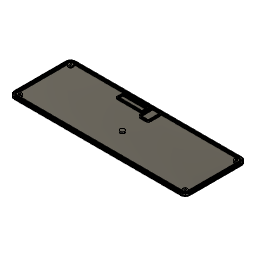
case-bottom (Autodesk Fusion 360 design; units mm, degrees)
Autodesk Fusion 360 part; units mm, degrees
sketch "triplejump-brd" plane through (0, -130, 0) normal (0, 0, 1) x (1, 0, 0)
  spline S0 degree 3 poles (13.4645, 139.4667) (14.4021, 138.529) (15.6739, 138.0022) (17, 138.0022) knots 0 0 0 0 1 1 1 1
  spline S1 degree 3 poles (352, 245.0022) (352, 246.3283) (351.4732, 247.6001) (350.5355, 248.5377) knots 0 0 0 0 1 1 1 1
  spline S2 degree 3 poles (350.5355, 248.5377) (349.5979, 249.4754) (348.3261, 250.0022) (347, 250.0022) knots 0 0 0 0 1 1 1 1
  spline S3 degree 3 poles (12, 143.0022) (12, 141.6761) (12.5268, 140.4043) (13.4645, 139.4667) knots 0 0 0 0 1 1 1 1
  line L0 (17, 138.0022) -> (347, 138.0022)
  spline S4 degree 3 poles (350.5355, 139.4667) (351.4732, 140.4043) (352, 141.6761) (352, 143.0022) knots 0 0 0 0 1 1 1 1
  spline S5 degree 3 poles (17, 250.0022) (15.6739, 250.0022) (14.4021, 249.4754) (13.4645, 248.5377) knots 0 0 0 0 1 1 1 1
  spline S6 degree 3 poles (13.4645, 248.5377) (12.5268, 247.6001) (12, 246.3283) (12, 245.0022) knots 0 0 0 0 1 1 1 1
  line L1 (176, 228.2522) -> (188, 228.2522)
  line L2 (12, 245.0022) -> (12, 143.0022)
  spline S7 degree 3 poles (347, 138.0022) (348.3261, 138.0022) (349.5979, 138.529) (350.5355, 139.4667) knots 0 0 0 0 1 1 1 1
  line L3 (352, 143.0022) -> (352, 245.0022)
  circle A0 centre (17, 245) radius 1.6
  circle A1 centre (17, 143) radius 1.6
  circle A2 centre (347, 143) radius 1.6
  circle A3 centre (347, 245) radius 1.6
  line L4 (166.8312, 244.5585) -> (121.6125, 244.5585)
  line L5 (121.6125, 237.0584) -> (166.8312, 237.0584)
  line L6 (166.8312, 237.0584) -> (166.8312, 244.5585)
  line L7 (121.6125, 244.5585) -> (121.6125, 237.0584)
  line L8 (176, 250.0022) -> (176, 228.2522)
  line L9 (188, 250.0022) -> (188, 228.2522)
  circle A4 centre (17, 245) radius 4.5
  circle A5 centre (17, 143) radius 4.5
  circle A6 centre (347, 143) radius 4.5
  circle A7 centre (347, 245) radius 4.5
  line L10 (277.3601, 186.5709) -> (278.3031, 184.453)
  line L11 (278.3031, 184.453) -> (262.316, 177.3352)
  line L12 (71.141, 245.3466) -> (87.1281, 238.2288)
  line L13 (54.2663, 211.342) -> (38.2793, 218.4598)
  line L14 (38.2793, 218.4598) -> (44.9905, 233.5333)
  line L15 (74.054, 205.1386) -> (55.2349, 213.5173)
  line L16 (89.0724, 195.8453) -> (73.0854, 202.9631)
  line L17 (95.7836, 210.9188) -> (89.0724, 195.8453)
  line L18 (316.9956, 238.0568) -> (334.3986, 245.8051)
  line L19 (297.7067, 234.5441) -> (315.1097, 242.2924)
  line L20 (315.1097, 242.2924) -> (316.9956, 238.0568)
  line L21 (281.7197, 227.4262) -> (280.7767, 229.5441)
  line L22 (296.7638, 236.6619) -> (297.7067, 234.5441)
  line L23 (280.7767, 229.5441) -> (296.7638, 236.6619)
  line L24 (264.3166, 219.6779) -> (281.7197, 227.4262)
  line L25 (265.2595, 217.56) -> (264.3166, 219.6779)
  line L26 (247.8565, 209.8117) -> (265.2595, 217.56)
  line L27 (348.8581, 213.3285) -> (332.8711, 206.2107)
  line L28 (332.8711, 206.2107) -> (330.9852, 210.4463)
  line L29 (313.5822, 202.698) -> (312.6393, 204.8158)
  line L30 (330.9852, 210.4463) -> (313.5822, 202.698)
  line L31 (312.6393, 204.8158) -> (293.8202, 196.437)
  line L32 (294.7632, 194.3192) -> (277.3601, 186.5709)
  line L33 (293.8202, 196.437) -> (294.7632, 194.3192)
  line L34 (83.663, 151.7163) -> (105.102, 167.2926)
  line L35 (105.102, 167.2926) -> (114.8005, 153.9439)
  line L36 (114.8005, 153.9439) -> (93.3615, 138.3676)
  line L37 (93.3615, 138.3676) -> (83.663, 151.7163)
  line L38 (258.898, 167.2926) -> (280.337, 151.7163)
  line L39 (249.1995, 153.9439) -> (258.898, 167.2926)
  line L40 (270.6385, 138.3676) -> (249.1995, 153.9439)
  line L41 (280.337, 151.7163) -> (270.6385, 138.3676)
  line L42 (176, 250.0022) -> (188, 250.0022)
  line L43 (347, 251.0022) -> (188, 251.0022)
  line L44 (176, 251.0022) -> (188, 251.0022)
  line L45 (17, 251.0022) -> (176, 251.0022)
  spline S8 degree 3 poles (17, 251.0022) (15.4091, 251.0022) (13.8823, 250.3698) (12.7574, 249.2448) knots 0 0 0 0 1 1 1 1
  spline S9 degree 3 poles (12.7574, 249.2448) (11.6324, 248.1199) (11, 246.5931) (11, 245.0022) knots 0 0 0 0 1 1 1 1
  line L46 (11, 245.0022) -> (11, 143.0022)
  spline S10 degree 3 poles (11, 143.0022) (11, 141.4113) (11.6324, 139.8845) (12.7574, 138.7596) knots 0 0 0 0 1 1 1 1
  spline S11 degree 3 poles (12.7574, 138.7596) (13.8823, 137.6346) (15.4091, 137.0022) (17, 137.0022) knots 0 0 0 0 1 1 1 1
  line L47 (17, 137.0022) -> (347, 137.0022)
  spline S12 degree 3 poles (347, 137.0022) (348.5909, 137.0022) (350.1177, 137.6346) (351.2426, 138.7596) knots 0 0 0 0 1 1 1 1
  spline S13 degree 3 poles (351.2426, 138.7596) (352.3676, 139.8845) (353, 141.4113) (353, 143.0022) knots 0 0 0 0 1 1 1 1
  line L48 (353, 143.0022) -> (353, 245.0022)
  spline S14 degree 3 poles (353, 245.0022) (353, 246.5931) (352.3676, 248.1199) (351.2426, 249.2448) knots 0 0 0 0 1 1 1 1
  spline S15 degree 3 poles (351.2426, 249.2448) (350.1177, 250.3698) (348.5909, 251.0022) (347, 251.0022) knots 0 0 0 0 1 1 1 1
  line L49 (347, 253.0022) -> (188, 253.0022)
  line L50 (176, 253.0022) -> (188, 253.0022)
  line L51 (17, 253.0022) -> (176, 253.0022)
  spline S16 degree 3 poles (17, 253.0022) (14.8794, 253.0022) (12.8426, 252.1585) (11.3431, 250.6591) knots 0 0 0 0 1 1 1 1
  spline S17 degree 3 poles (11.3431, 250.6591) (9.8437, 249.1596) (9, 247.1228) (9, 245.0022) knots 0 0 0 0 1 1 1 1
  line L52 (9, 245.0022) -> (9, 143.0022)
  spline S18 degree 3 poles (9, 143.0022) (9, 140.8816) (9.8437, 138.8448) (11.3431, 137.3453) knots 0 0 0 0 1 1 1 1
  spline S19 degree 3 poles (11.3431, 137.3453) (12.8426, 135.8459) (14.8794, 135.0022) (17, 135.0022) knots 0 0 0 0 1 1 1 1
  line L53 (17, 135.0022) -> (347, 135.0022)
  spline S20 degree 3 poles (347, 135.0022) (349.1206, 135.0022) (351.1574, 135.8459) (352.6569, 137.3453) knots 0 0 0 0 1 1 1 1
  spline S21 degree 3 poles (352.6569, 137.3453) (354.1563, 138.8448) (355, 140.8816) (355, 143.0022) knots 0 0 0 0 1 1 1 1
  line L54 (355, 143.0022) -> (355, 245.0022)
  spline S22 degree 3 poles (355, 245.0022) (355, 247.1228) (354.1563, 249.1596) (352.6569, 250.6591) knots 0 0 0 0 1 1 1 1
  spline S23 degree 3 poles (352.6569, 250.6591) (351.1574, 252.1585) (349.1206, 253.0022) (347, 253.0022) knots 0 0 0 0 1 1 1 1
  line L55 (347, 255.0022) -> (188, 255.0022)
  line L56 (176, 255.0022) -> (188, 255.0022)
  line L57 (17, 255.0022) -> (176, 255.0022)
  spline S24 degree 3 poles (17, 255.0022) (14.3498, 255.0022) (11.8029, 253.9473) (9.9289, 252.0733) knots 0 0 0 0 1 1 1 1
  spline S25 degree 3 poles (9.9289, 252.0733) (8.0549, 250.1993) (7, 247.6524) (7, 245.0022) knots 0 0 0 0 1 1 1 1
  line L58 (7, 245.0022) -> (7, 143.0022)
  spline S26 degree 3 poles (7, 143.0022) (7, 140.352) (8.0549, 137.8051) (9.9289, 135.9311) knots 0 0 0 0 1 1 1 1
  spline S27 degree 3 poles (9.9289, 135.9311) (11.8029, 134.0571) (14.3498, 133.0022) (17, 133.0022) knots 0 0 0 0 1 1 1 1
  line L59 (17, 133.0022) -> (347, 133.0022)
  spline S28 degree 3 poles (347, 133.0022) (349.6502, 133.0022) (352.1971, 134.0571) (354.0711, 135.9311) knots 0 0 0 0 1 1 1 1
  spline S29 degree 3 poles (354.0711, 135.9311) (355.9451, 137.8051) (357, 140.352) (357, 143.0022) knots 0 0 0 0 1 1 1 1
  line L60 (357, 143.0022) -> (357, 245.0022)
  spline S30 degree 3 poles (357, 245.0022) (357, 247.6524) (355.9451, 250.1993) (354.0711, 252.0733) knots 0 0 0 0 1 1 1 1
  spline S31 degree 3 poles (354.0711, 252.0733) (352.1971, 253.9473) (349.6502, 255.0022) (347, 255.0022) knots 0 0 0 0 1 1 1 1
  line L61 (55.2349, 213.5173) -> (54.2663, 211.342)
  line L62 (71.141, 245.3466) -> (62.3935, 225.785)
  line L63 (87.1281, 238.2288) -> (78.3805, 218.6671)
  line L64 (74.054, 205.1386) -> (73.0854, 202.9631)
  line L65 (44.9905, 233.5333) -> (62.3935, 225.785)
  line L66 (78.3805, 218.6671) -> (95.7836, 210.9188)
  line L67 (247.8565, 209.8117) -> (262.316, 177.3352)
  line L68 (348.8581, 213.3285) -> (334.3986, 245.8051)
  circle A8 centre (182, 183.1272) radius 4.5
  line L69 (350.1754, 143) -> (348.5877, 145.75)
  line L70 (348.5877, 145.75) -> (345.4123, 145.75)
  line L71 (345.4123, 145.75) -> (343.8246, 143)
  line L72 (343.8246, 143) -> (345.4123, 140.25)
  line L73 (345.4123, 140.25) -> (348.5877, 140.25)
  line L74 (348.5877, 140.25) -> (350.1754, 143)
  line L75 (20.1754, 245) -> (18.5877, 247.75)
  line L76 (15.4123, 247.75) -> (13.8246, 245)
  line L77 (18.5877, 247.75) -> (15.4123, 247.75)
  line L78 (18.5877, 242.25) -> (20.1754, 245)
  line L79 (15.4123, 242.25) -> (18.5877, 242.25)
  line L80 (13.8246, 245) -> (15.4123, 242.25)
  line L81 (15.4123, 140.25) -> (18.5877, 140.25)
  line L82 (18.5877, 145.75) -> (15.4123, 145.75)
  line L83 (20.1754, 143) -> (18.5877, 145.75)
  line L84 (15.4123, 145.75) -> (13.8246, 143)
  line L85 (13.8246, 143) -> (15.4123, 140.25)
  line L86 (18.5877, 140.25) -> (20.1754, 143)
  line L87 (348.5877, 242.25) -> (350.1754, 245)
  line L88 (348.5877, 247.75) -> (345.4123, 247.75)
  line L89 (345.4123, 247.75) -> (343.8246, 245)
  line L90 (345.4123, 242.25) -> (348.5877, 242.25)
  line L91 (350.1754, 245) -> (348.5877, 247.75)
  line L92 (343.8246, 245) -> (345.4123, 242.25)
  line L93 (174, 249.0022) -> (174, 228.2522)
  line L94 (176, 226.2522) -> (188, 226.2522)
  line L95 (190, 249.0022) -> (190, 228.2522)
  line L96 (121.6125, 236.0584) -> (166.8312, 236.0584)
  line L97 (167.8312, 237.0584) -> (167.8312, 244.5585)
  line L98 (166.8312, 245.5585) -> (121.6125, 245.5585)
  line L99 (120.6125, 244.5585) -> (120.6125, 237.0584)
  line L100 (44.8904, 235.7672) -> (60.4708, 228.8303)
  line L101 (69.7228, 247.0745) -> (61.7904, 229.3357)
  line L102 (71.0424, 247.5798) -> (88.8566, 239.6484)
  line L103 (89.3627, 238.3267) -> (81.433, 220.5938)
  line L104 (81.9391, 219.272) -> (97.5106, 212.3391)
  line L105 (98.0174, 211.0188) -> (90.4928, 194.1182)
  line L106 (89.1725, 193.6114) -> (71.3584, 201.5428)
  line L107 (71.0067, 203.2114) -> (70.8516, 202.8631)
  line L108 (70.4998, 204.5317) -> (57.1621, 210.47)
  line L109 (55.8418, 209.9632) -> (55.6867, 209.6149)
  line L110 (54.3664, 209.1081) -> (36.5523, 217.0395)
  line L111 (36.0455, 218.3598) -> (43.5701, 235.2604)
  line L112 (116.785, 152.9136) -> (93.7281, 136.1617)
  line L113 (92.3313, 136.383) -> (81.4572, 151.3498)
  line L114 (81.6785, 152.7466) -> (104.7354, 169.4985)
  line L115 (106.1322, 169.2772) -> (117.0063, 154.3104)
  line L116 (299.6339, 237.5914) -> (315.2098, 244.5263)
  line L117 (316.5301, 244.0195) -> (317.6025, 241.6109)
  line L118 (318.9227, 241.1041) -> (334.4987, 248.0389)
  line L119 (351.0919, 213.2285) -> (335.8189, 247.5321)
  line L120 (350.5851, 211.9082) -> (332.771, 203.9768)
  line L121 (331.4507, 204.4836) -> (330.3784, 206.8922)
  line L122 (329.0581, 207.399) -> (313.4821, 200.4641)
  line L123 (312.1618, 200.9709) -> (312.0324, 201.2617)
  line L124 (310.7121, 201.7685) -> (297.3743, 195.8301)
  line L125 (296.8675, 194.5099) -> (296.997, 194.2191)
  line L126 (296.4902, 192.8988) -> (280.9142, 185.964)
  line L127 (280.4074, 184.6437) -> (280.5369, 184.353)
  line L128 (280.0301, 183.0327) -> (262.2159, 175.1013)
  line L129 (245.6227, 209.9118) -> (260.8957, 175.6081)
  line L130 (246.1295, 211.2321) -> (261.7054, 218.1669)
  line L131 (262.2122, 219.4872) -> (262.0828, 219.7779)
  line L132 (262.5896, 221.0982) -> (278.1656, 228.0331)
  line L133 (278.6724, 229.3534) -> (278.5429, 229.6441)
  line L134 (279.0497, 230.9644) -> (296.8639, 238.8958)
  line L135 (298.1841, 238.389) -> (298.3136, 238.0982)
  line L136 (270.2719, 136.1617) -> (247.215, 152.9136)
  line L137 (246.9937, 154.3104) -> (257.8678, 169.2772)
  line L138 (259.2646, 169.4985) -> (282.3215, 152.7466)
  line L139 (282.5428, 151.3498) -> (271.6687, 136.383)
  line L140 (172, 249.0022) -> (172, 228.2522)
  line L141 (176, 224.2522) -> (188, 224.2522)
  line L142 (192, 249.0022) -> (192, 228.2522)
  arc A9 (174, 228.2522) -> (176, 226.2522) centre (176, 228.2522) ccw
  arc A10 (188, 226.2522) -> (190, 228.2522) centre (188, 228.2522) ccw
  arc A11 (174, 249.0022) -> (173, 250.0022) centre (173, 249.0022) ccw
  arc A12 (173, 250.0022) -> (172, 249.0022) centre (173, 249.0022) ccw
  arc A13 (191, 250.0022) -> (190, 249.0022) centre (191, 249.0022) ccw
  arc A14 (192, 249.0022) -> (191, 250.0022) centre (191, 249.0022) ccw
  arc A15 (172, 228.2522) -> (176, 224.2522) centre (176, 228.2522) ccw
  arc A16 (188, 224.2522) -> (192, 228.2522) centre (188, 228.2522) ccw
  line L143 (119.6125, 234.0584) -> (168.8312, 234.0584)
  line L144 (169.8312, 235.0584) -> (169.8312, 246.5585)
  line L145 (168.8312, 247.5585) -> (119.6125, 247.5585)
  line L146 (118.6125, 246.5585) -> (118.6125, 235.0584)
  line L147 (68.7121, 249.7137) -> (60.7798, 231.9749)
  line L148 (43.8768, 238.4077) -> (59.4601, 231.4696)
  line L149 (33.4049, 217.3462) -> (42.5565, 237.9009)
  line L150 (55.38, 206.4676) -> (33.9117, 216.0259)
  line L151 (56.8554, 207.3227) -> (56.7003, 206.9744)
  line L152 (67.8593, 203.5181) -> (58.1757, 207.8295)
  line L153 (68.3661, 202.1978) -> (68.211, 201.8495)
  line L154 (90.1861, 190.9709) -> (68.7178, 200.5292)
  line L155 (100.658, 212.0324) -> (91.5064, 191.4777)
  line L156 (84.5826, 220.2843) -> (100.1512, 213.3527)
  line L157 (92.0062, 239.339) -> (84.0765, 221.6061)
  line L158 (70.0318, 250.2191) -> (91.5001, 240.6607)
  line L159 (259.949, 222.1118) -> (275.525, 229.0467)
  line L160 (276.0318, 230.367) -> (275.9024, 230.6577)
  line L161 (276.4092, 231.978) -> (297.8775, 241.5363)
  line L162 (299.1978, 241.0295) -> (299.3272, 240.7388)
  line L163 (300.6475, 240.232) -> (316.2234, 247.1668)
  line L164 (317.5437, 246.66) -> (318.6161, 244.2515)
  line L165 (319.9364, 243.7446) -> (335.5123, 250.6795)
  line L166 (353.7325, 212.2149) -> (336.8326, 250.1727)
  line L167 (353.2257, 210.8946) -> (331.7574, 201.3363)
  line L168 (330.4371, 201.8431) -> (329.3647, 204.2516)
  line L169 (328.0445, 204.7584) -> (312.4685, 197.8236)
  line L170 (311.1482, 198.3304) -> (311.0188, 198.6211)
  line L171 (309.6985, 199.1279) -> (300.0149, 194.8165)
  line L172 (299.5081, 193.4962) -> (299.6375, 193.2055)
  line L173 (299.1307, 191.8852) -> (283.5548, 184.9504)
  line L174 (283.048, 183.6301) -> (283.1774, 183.3394)
  line L175 (282.6706, 182.0191) -> (261.2023, 172.4608)
  line L176 (242.9821, 210.9254) -> (259.882, 172.9676)
  line L177 (243.4889, 212.2457) -> (259.0648, 219.1805)
  line L178 (259.5717, 220.5008) -> (259.4422, 220.7915)
  line L179 (119.5786, 152.4712) -> (93.2856, 133.3681)
  line L180 (91.8888, 133.5894) -> (78.6636, 151.7922)
  line L181 (78.8849, 153.189) -> (105.1779, 172.2921)
  line L182 (106.5747, 172.0708) -> (119.7999, 153.868)
  line L183 (285.3364, 151.7922) -> (272.1112, 133.5894)
  line L184 (270.7144, 133.3681) -> (244.4214, 152.4712)
  line L185 (244.2001, 153.868) -> (257.4253, 172.0708)
  line L186 (258.8221, 172.2921) -> (285.1151, 153.189)
  arc A17 (43.8768, 238.4077) -> (42.5565, 237.9009) centre (43.47, 237.4942) ccw
  arc A18 (44.8904, 235.7672) -> (43.5701, 235.2604) centre (44.4836, 234.8536) ccw
  arc A19 (59.4601, 231.4696) -> (60.7798, 231.9749) centre (59.8669, 232.3831) ccw
  arc A20 (60.4708, 228.8303) -> (61.7904, 229.3357) centre (60.8775, 229.7439) ccw
  arc A21 (71.0424, 247.5798) -> (69.7228, 247.0745) centre (70.6357, 246.6663) ccw
  arc A22 (70.0318, 250.2191) -> (68.7121, 249.7137) centre (69.625, 249.3055) ccw
  arc A23 (89.3627, 238.3267) -> (88.8566, 239.6484) centre (88.4498, 238.7349) ccw
  arc A24 (92.0062, 239.339) -> (91.5001, 240.6607) centre (91.0934, 239.7472) ccw
  arc A25 (84.0765, 221.6061) -> (84.5826, 220.2843) centre (84.9894, 221.1978) ccw
  arc A26 (81.433, 220.5938) -> (81.9391, 219.272) centre (82.3458, 220.1855) ccw
  arc A27 (100.658, 212.0324) -> (100.1512, 213.3527) centre (99.7444, 212.4392) ccw
  arc A28 (98.0174, 211.0188) -> (97.5106, 212.3391) centre (97.1039, 211.4256) ccw
  arc A29 (89.1725, 193.6114) -> (90.4928, 194.1182) centre (89.5793, 194.525) ccw
  arc A30 (90.1861, 190.9709) -> (91.5064, 191.4777) centre (90.5929, 191.8844) ccw
  arc A31 (70.8516, 202.8631) -> (71.3584, 201.5428) centre (71.7651, 202.4563) ccw
  arc A32 (71.0067, 203.2114) -> (70.4998, 204.5317) centre (70.0931, 203.6181) ccw
  arc A33 (68.3661, 202.1978) -> (67.8593, 203.5181) centre (67.4525, 202.6045) ccw
  arc A34 (68.211, 201.8495) -> (68.7178, 200.5292) centre (69.1246, 201.4427) ccw
  arc A35 (57.1621, 210.47) -> (55.8418, 209.9632) centre (56.7553, 209.5565) ccw
  arc A36 (54.3664, 209.1081) -> (55.6867, 209.6149) centre (54.7732, 210.0217) ccw
  arc A37 (58.1757, 207.8295) -> (56.8554, 207.3227) centre (57.7689, 206.9159) ccw
  arc A38 (55.38, 206.4676) -> (56.7003, 206.9744) centre (55.7868, 207.3811) ccw
  arc A39 (36.0455, 218.3598) -> (36.5523, 217.0395) centre (36.959, 217.953) ccw
  arc A40 (33.4049, 217.3462) -> (33.9117, 216.0259) centre (34.3185, 216.9394) ccw
  arc A41 (121.6125, 245.5585) -> (120.6125, 244.5585) centre (121.6125, 244.5585) ccw
  arc A42 (120.6125, 237.0584) -> (121.6125, 236.0584) centre (121.6125, 237.0584) ccw
  arc A43 (119.6125, 247.5585) -> (118.6125, 246.5585) centre (119.6125, 246.5585) ccw
  arc A44 (118.6125, 235.0584) -> (119.6125, 234.0584) centre (119.6125, 235.0584) ccw
  arc A45 (168.8312, 234.0584) -> (169.8312, 235.0584) centre (168.8312, 235.0584) ccw
  arc A46 (166.8312, 236.0584) -> (167.8312, 237.0584) centre (166.8312, 237.0584) ccw
  arc A47 (167.8312, 244.5585) -> (166.8312, 245.5585) centre (166.8312, 244.5585) ccw
  arc A48 (169.8312, 246.5585) -> (168.8312, 247.5585) centre (168.8312, 246.5585) ccw
  arc A49 (243.4889, 212.2457) -> (242.9821, 210.9254) centre (243.8957, 211.3321) ccw
  arc A50 (246.1295, 211.2321) -> (245.6227, 209.9118) centre (246.5362, 210.3185) ccw
  arc A51 (259.0648, 219.1805) -> (259.5717, 220.5008) centre (258.6581, 220.0941) ccw
  arc A52 (259.949, 222.1118) -> (259.4422, 220.7915) centre (260.3558, 221.1983) ccw
  arc A53 (261.7054, 218.1669) -> (262.2122, 219.4872) centre (261.2987, 219.0805) ccw
  arc A54 (262.5896, 221.0982) -> (262.0828, 219.7779) centre (262.9963, 220.1847) ccw
  arc A55 (275.525, 229.0467) -> (276.0318, 230.367) centre (275.1183, 229.9602) ccw
  arc A56 (276.4092, 231.978) -> (275.9024, 230.6577) centre (276.8159, 231.0645) ccw
  arc A57 (278.1656, 228.0331) -> (278.6724, 229.3534) centre (277.7588, 228.9466) ccw
  arc A58 (279.0497, 230.9644) -> (278.5429, 229.6441) centre (279.4565, 230.0509) ccw
  arc A59 (299.1978, 241.0295) -> (297.8775, 241.5363) centre (298.2842, 240.6228) ccw
  arc A60 (298.1841, 238.389) -> (296.8639, 238.8958) centre (297.2706, 237.9822) ccw
  arc A61 (298.3136, 238.0982) -> (299.6339, 237.5914) centre (299.2271, 238.505) ccw
  arc A62 (299.3272, 240.7388) -> (300.6475, 240.232) centre (300.2408, 241.1455) ccw
  arc A63 (316.5301, 244.0195) -> (315.2098, 244.5263) centre (315.6166, 243.6127) ccw
  arc A64 (317.5437, 246.66) -> (316.2234, 247.1668) centre (316.6302, 246.2533) ccw
  arc A65 (318.6161, 244.2515) -> (319.9364, 243.7446) centre (319.5296, 244.6582) ccw
  arc A66 (317.6025, 241.6109) -> (318.9227, 241.1041) centre (318.516, 242.0176) ccw
  arc A67 (336.8326, 250.1727) -> (335.5123, 250.6795) centre (335.919, 249.7659) ccw
  arc A68 (335.8189, 247.5321) -> (334.4987, 248.0389) centre (334.9054, 247.1254) ccw
  arc A69 (353.2257, 210.8946) -> (353.7325, 212.2149) centre (352.8189, 211.8081) ccw
  arc A70 (350.5851, 211.9082) -> (351.0919, 213.2285) centre (350.1784, 212.8217) ccw
  arc A71 (331.4507, 204.4836) -> (332.771, 203.9768) centre (332.3642, 204.8904) ccw
  arc A72 (330.4371, 201.8431) -> (331.7574, 201.3363) centre (331.3506, 202.2498) ccw
  arc A73 (330.3784, 206.8922) -> (329.0581, 207.399) centre (329.4648, 206.4854) ccw
  arc A74 (329.3647, 204.2516) -> (328.0445, 204.7584) centre (328.4512, 203.8449) ccw
  arc A75 (312.1618, 200.9709) -> (313.4821, 200.4641) centre (313.0754, 201.3777) ccw
  arc A76 (311.1482, 198.3304) -> (312.4685, 197.8236) centre (312.0618, 198.7371) ccw
  arc A77 (312.0324, 201.2617) -> (310.7121, 201.7685) centre (311.1188, 200.855) ccw
  arc A78 (311.0188, 198.6211) -> (309.6985, 199.1279) centre (310.1052, 198.2144) ccw
  arc A79 (297.3743, 195.8301) -> (296.8675, 194.5099) centre (297.7811, 194.9166) ccw
  arc A80 (296.4902, 192.8988) -> (296.997, 194.2191) centre (296.0834, 193.8124) ccw
  arc A81 (300.0149, 194.8165) -> (299.5081, 193.4962) centre (300.4216, 193.903) ccw
  arc A82 (299.1307, 191.8852) -> (299.6375, 193.2055) centre (298.724, 192.7988) ccw
  arc A83 (280.9142, 185.964) -> (280.4074, 184.6437) centre (281.321, 185.0504) ccw
  arc A84 (280.0301, 183.0327) -> (280.5369, 184.353) centre (279.6233, 183.9462) ccw
  arc A85 (283.5548, 184.9504) -> (283.048, 183.6301) centre (283.9615, 184.0368) ccw
  arc A86 (282.6706, 182.0191) -> (283.1774, 183.3394) centre (282.2639, 182.9326) ccw
  arc A87 (260.8957, 175.6081) -> (262.2159, 175.1013) centre (261.8092, 176.0149) ccw
  arc A88 (259.882, 172.9676) -> (261.2023, 172.4608) centre (260.7956, 173.3743) ccw
  line L187 (17, 250.0022) -> (347, 250.0022)
  arc A89 (259.2646, 169.4985) -> (257.8678, 169.2772) centre (258.6768, 168.6894) ccw
  arc A90 (258.8221, 172.2921) -> (257.4253, 172.0708) centre (258.2343, 171.4831) ccw
  arc A91 (285.3364, 151.7922) -> (285.1151, 153.189) centre (284.5274, 152.38) ccw
  arc A92 (282.5428, 151.3498) -> (282.3215, 152.7466) centre (281.7338, 151.9376) ccw
  arc A93 (270.2719, 136.1617) -> (271.6687, 136.383) centre (270.8597, 136.9708) ccw
  arc A94 (270.7144, 133.3681) -> (272.1112, 133.5894) centre (271.3022, 134.1771) ccw
  arc A95 (246.9937, 154.3104) -> (247.215, 152.9136) centre (247.8027, 153.7226) ccw
  arc A96 (244.2001, 153.868) -> (244.4214, 152.4712) centre (245.0091, 153.2802) ccw
  arc A97 (81.6785, 152.7466) -> (81.4572, 151.3498) centre (82.2662, 151.9376) ccw
  arc A98 (92.3313, 136.383) -> (93.7281, 136.1617) centre (93.1403, 136.9708) ccw
  arc A99 (106.1322, 169.2772) -> (104.7354, 169.4985) centre (105.3232, 168.6894) ccw
  arc A100 (116.785, 152.9136) -> (117.0063, 154.3104) centre (116.1973, 153.7226) ccw
  arc A101 (106.5747, 172.0708) -> (105.1779, 172.2921) centre (105.7657, 171.4831) ccw
  arc A102 (119.5786, 152.4712) -> (119.7999, 153.868) centre (118.9909, 153.2802) ccw
  arc A103 (78.8849, 153.189) -> (78.6636, 151.7922) centre (79.4726, 152.38) ccw
  arc A104 (91.8888, 133.5894) -> (93.2856, 133.3681) centre (92.6978, 134.1771) ccw
  line L188 (175.5, 255.0022) -> (188.5, 255.0022)
  line L189 (188.5, 255.0022) -> (188.5, 250.0022)
  line L190 (188.5, 250.0022) -> (175.5, 250.0022)
  line L191 (175.5, 250.0022) -> (175.5, 255.0022)
  point P0 (182, 183.1272)
  point P1 (347, 143)
  point P2 (17, 245)
  point P3 (17, 143)
  point P4 (347, 245)
  point P5 (182, 255.0022)
  point P6 (182, 255.0022)
  dimension "d90" = 3.1754
  dimension "d91" = 3.1754
  dimension "d92" = 3.1754
  dimension "d93" = 3.1754
  dimension "d112" = 2
  dimension "d113" = 2
  dimension "d114" = 1
  dimension "d115" = 1
  dimension "d116" = 1
  dimension "d117" = 1
  dimension "d118" = 4
  dimension "d119" = 4
  dimension "d125" = 1
  dimension "d126" = 1
  dimension "d127" = 1
  dimension "d128" = 1
  dimension "d129" = 1
  dimension "d130" = 1
  dimension "d131" = 1
  dimension "d132" = 1
  dimension "d133" = 1
  dimension "d134" = 1
  dimension "d135" = 1
  dimension "d136" = 1
  dimension "d137" = 1
  dimension "d138" = 1
  dimension "d139" = 1
  dimension "d140" = 1
  dimension "d141" = 1
  dimension "d142" = 1
  dimension "d143" = 1
  dimension "d144" = 1
  dimension "d145" = 1
  dimension "d146" = 1
  dimension "d147" = 1
  dimension "d148" = 1
  dimension "d149" = 1
  dimension "d150" = 1
  dimension "d151" = 1
  dimension "d152" = 1
  dimension "d153" = 1
  dimension "d154" = 1
  dimension "d155" = 1
  dimension "d156" = 1
  dimension "d157" = 1
  dimension "d158" = 1
  dimension "d159" = 1
  dimension "d160" = 1
  dimension "d161" = 1
  dimension "d162" = 1
  dimension "d163" = 1
  dimension "d164" = 1
  dimension "d165" = 1
  dimension "d166" = 1
  dimension "d167" = 1
  dimension "d168" = 1
  dimension "d169" = 1
  dimension "d170" = 1
  dimension "d171" = 1
  dimension "d172" = 1
  dimension "d173" = 1
  dimension "d174" = 1
  dimension "d175" = 1
  dimension "d176" = 1
  dimension "d177" = 1
  dimension "d178" = 1
  dimension "d179" = 1
  dimension "d180" = 1
  dimension "d181" = 1
  dimension "d182" = 1
  dimension "d183" = 1
  dimension "d184" = 1
  dimension "d185" = 1
  dimension "d186" = 1
  dimension "d187" = 1
  dimension "d188" = 1
  dimension "d189" = 1
  dimension "d190" = 1
  dimension "d191" = 1
  dimension "d192" = 1
  dimension "d193" = 1
  dimension "d194" = 1
  dimension "d195" = 1
  dimension "d196" = 1
  dimension "d197" = 1
  dimension "d198" = 1
  dimension "d199" = 1
  dimension "d200" = 1
  dimension "d201" = 1
  dimension "d202" = 1
  dimension "d203" = 1
  dimension "d204" = 1
  dimension "d205" = 1
  dimension "d206" = 1
  dimension "d207" = 1
  dimension "d208" = 1
  dimension "d209" = 1
  dimension "d210" = 1
  dimension "d211" = 1
  dimension "d212" = 1
  constraint concentric A1 A5
  constraint concentric A3 A7
  constraint perpendicular L9 L42
  constraint perpendicular L13 L61
  constraint perpendicular L16 L64
  constraint perpendicular L17 L66
  constraint coincident P0 A8.centre
  constraint tangent L93 A9
  constraint tangent L94 A9
  constraint tangent L94 A10
  constraint tangent L95 A10
  constraint tangent L93 A11
  constraint tangent L140 A12
  constraint coincident A11.end A12.start
  constraint tangent L95 A13
  constraint tangent L142 A14
  constraint coincident A13.start A14.end
  constraint tangent L141 A15
  constraint tangent L140 A15
  constraint tangent L141 A16
  constraint tangent L142 A16
  constraint tangent L148 A17
  constraint tangent L149 A17
  constraint tangent L111 A18
  constraint tangent L100 A18
  constraint tangent L148 A19
  constraint tangent L147 A19
  constraint tangent L100 A20
  constraint tangent L101 A20
  constraint tangent L101 A21
  constraint tangent L102 A21
  constraint tangent L147 A22
  constraint tangent L158 A22
  constraint tangent L102 A23
  constraint tangent L103 A23
  constraint tangent L158 A24
  constraint tangent L157 A24
  constraint tangent L157 A25
  constraint tangent L156 A25
  constraint tangent L103 A26
  constraint tangent L104 A26
  constraint tangent L156 A27
  constraint tangent L155 A27
  constraint tangent L104 A28
  constraint tangent L105 A28
  constraint tangent L105 A29
  constraint tangent L106 A29
  constraint tangent L154 A30
  constraint tangent L155 A30
  constraint tangent L106 A31
  constraint tangent L107 A31
  constraint tangent L108 A32
  constraint tangent L107 A32
  constraint tangent L152 A33
  constraint tangent L153 A33
  constraint tangent L153 A34
  constraint tangent L154 A34
  constraint tangent L108 A35
  constraint tangent L109 A35
  constraint tangent L109 A36
  constraint tangent L110 A36
  constraint tangent L152 A37
  constraint tangent L151 A37
  constraint tangent L151 A38
  constraint tangent L150 A38
  constraint tangent L110 A39
  constraint tangent L111 A39
  constraint tangent L150 A40
  constraint tangent L149 A40
  constraint tangent L98 A41
  constraint tangent L99 A41
  constraint tangent L99 A42
  constraint tangent L96 A42
  constraint tangent L146 A43
  constraint tangent L145 A43
  constraint tangent L146 A44
  constraint tangent L143 A44
  constraint tangent L143 A45
  constraint tangent L144 A45
  constraint tangent L96 A46
  constraint tangent L97 A46
  constraint tangent L98 A47
  constraint tangent L97 A47
  constraint tangent L145 A48
  constraint tangent L144 A48
  constraint tangent L176 A49
  constraint tangent L177 A49
  constraint tangent L129 A50
  constraint tangent L130 A50
  constraint tangent L177 A51
  constraint tangent L178 A51
  constraint tangent L178 A52
  constraint tangent L159 A52
  constraint tangent L130 A53
  constraint tangent L131 A53
  constraint tangent L131 A54
  constraint tangent L132 A54
  constraint tangent L159 A55
  constraint tangent L160 A55
  constraint tangent L160 A56
  constraint tangent L161 A56
  constraint tangent L132 A57
  constraint tangent L133 A57
  constraint tangent L133 A58
  constraint tangent L134 A58
  constraint tangent L161 A59
  constraint tangent L162 A59
  constraint tangent L134 A60
  constraint tangent L135 A60
  constraint tangent L135 A61
  constraint tangent L116 A61
  constraint tangent L162 A62
  constraint tangent L163 A62
  constraint tangent L116 A63
  constraint tangent L117 A63
  constraint tangent L163 A64
  constraint tangent L164 A64
  constraint tangent L164 A65
  constraint tangent L165 A65
  constraint tangent L117 A66
  constraint tangent L118 A66
  constraint tangent L165 A67
  constraint tangent L166 A67
  constraint tangent L118 A68
  constraint tangent L119 A68
  constraint tangent L166 A69
  constraint tangent L167 A69
  constraint tangent L119 A70
  constraint tangent L120 A70
  constraint tangent L120 A71
  constraint tangent L121 A71
  constraint tangent L167 A72
  constraint tangent L168 A72
  constraint tangent L121 A73
  constraint tangent L122 A73
  constraint tangent L168 A74
  constraint tangent L169 A74
  constraint tangent L122 A75
  constraint tangent L123 A75
  constraint tangent L170 A76
  constraint tangent L169 A76
  constraint tangent L123 A77
  constraint tangent L124 A77
  constraint tangent L171 A78
  constraint tangent L170 A78
  constraint tangent L124 A79
  constraint tangent L125 A79
  constraint tangent L126 A80
  constraint tangent L125 A80
  constraint tangent L171 A81
  constraint tangent L172 A81
  constraint tangent L173 A82
  constraint tangent L172 A82
  constraint tangent L126 A83
  constraint tangent L127 A83
  constraint tangent L127 A84
  constraint tangent L128 A84
  constraint tangent L173 A85
  constraint tangent L174 A85
  constraint tangent L175 A86
  constraint tangent L174 A86
  constraint tangent L128 A87
  constraint tangent L129 A87
  constraint tangent L175 A88
  constraint tangent L176 A88
  constraint tangent L137 A89
  constraint tangent L138 A89
  constraint tangent L185 A90
  constraint tangent L186 A90
  constraint tangent L186 A91
  constraint tangent L183 A91
  constraint tangent L138 A92
  constraint tangent L139 A92
  constraint tangent L139 A93
  constraint tangent L136 A93
  constraint tangent L183 A94
  constraint tangent L184 A94
  constraint tangent L137 A95
  constraint tangent L136 A95
  constraint tangent L185 A96
  constraint tangent L184 A96
  constraint tangent L114 A97
  constraint tangent L113 A97
  constraint tangent L113 A98
  constraint tangent L112 A98
  constraint tangent L114 A99
  constraint tangent L115 A99
  constraint tangent L115 A100
  constraint tangent L112 A100
  constraint tangent L181 A101
  constraint tangent L182 A101
  constraint tangent L182 A102
  constraint tangent L179 A102
  constraint tangent L181 A103
  constraint tangent L180 A103
  constraint tangent L180 A104
  constraint tangent L179 A104
  constraint midpoint L56 P6
  constraint horizontal L188
  constraint vertical L189
  constraint horizontal L190
  constraint vertical L191
  constraint midpoint L188 P6
  measures "d90" distance of L69.start P1
  measures "d91" distance of L75.start P2
  measures "d92" distance of L83.start P3
  measures "d93" distance of L87.end P4
  measures "d112" radius of A9
  measures "d113" radius of A10
  measures "d114" radius of A11
  measures "d115" radius of A12
  measures "d116" radius of A13
  measures "d117" radius of A14
  measures "d118" radius of A15
  measures "d119" radius of A16
  measures "d125" radius of A17
  measures "d126" radius of A18
  measures "d127" radius of A19
  measures "d128" radius of A20
  measures "d129" radius of A21
  measures "d130" radius of A22
  measures "d131" radius of A23
  measures "d132" radius of A24
  measures "d133" radius of A25
  measures "d134" radius of A26
  measures "d135" radius of A27
  measures "d136" radius of A28
  measures "d137" radius of A29
  measures "d138" radius of A30
  measures "d139" radius of A31
  measures "d140" radius of A32
  measures "d141" radius of A33
  measures "d142" radius of A34
  measures "d143" radius of A35
  measures "d144" radius of A36
  measures "d145" radius of A37
  measures "d146" radius of A38
  measures "d147" radius of A39
  measures "d148" radius of A40
  measures "d149" radius of A41
  measures "d150" radius of A42
  measures "d151" radius of A43
  measures "d152" radius of A44
  measures "d153" radius of A45
  measures "d154" radius of A46
  measures "d155" radius of A47
  measures "d156" radius of A48
  measures "d157" radius of A49
  measures "d158" radius of A50
  measures "d159" radius of A51
  measures "d160" radius of A52
  measures "d161" radius of A53
  measures "d162" radius of A54
  measures "d163" radius of A55
  measures "d164" radius of A56
  measures "d165" radius of A57
  measures "d166" radius of A58
  measures "d167" radius of A59
  measures "d168" radius of A60
  measures "d169" radius of A61
  measures "d170" radius of A62
  measures "d171" radius of A63
  measures "d172" radius of A64
  measures "d173" radius of A65
  measures "d174" radius of A66
  measures "d175" radius of A67
  measures "d176" radius of A68
  measures "d177" radius of A69
  measures "d178" radius of A70
  measures "d179" radius of A71
  measures "d180" radius of A72
  measures "d181" radius of A73
  measures "d182" radius of A74
  measures "d183" radius of A75
  measures "d184" radius of A76
  measures "d185" radius of A77
  measures "d186" radius of A78
  measures "d187" radius of A79
  measures "d188" radius of A80
  measures "d189" radius of A81
  measures "d190" radius of A82
  measures "d191" radius of A83
  measures "d192" radius of A84
  measures "d193" radius of A85
  measures "d194" radius of A86
  measures "d195" radius of A87
  measures "d196" radius of A88
  measures "d197" radius of A89
  measures "d198" radius of A90
  measures "d199" radius of A91
  measures "d200" radius of A92
  measures "d201" radius of A93
  measures "d202" radius of A94
  measures "d203" radius of A95
  measures "d204" radius of A96
  measures "d205" radius of A97
  measures "d206" radius of A98
  measures "d207" radius of A99
  measures "d208" radius of A100
  measures "d209" radius of A101
  measures "d210" radius of A102
  measures "d211" radius of A103
  measures "d212" radius of A104
extrude "Extrude14" add sketch "triplejump-brd" along normal blind 2 contours S0 S3 L0 S4 S5 S6 L2 S7 L3 L140 L141 L142 A12 A14 A15 A16 L147 L148 L149 L150 L151 L152 L153 L154 L155 L156 L157 L158 L159 L160 L161 L162 L163 L164 L165 L167 L168 L169 L170 L171 L172 L173 L174 L175 L176 L177 L178 L179 L180 L181 L182 L183 L184 L185 L186 A17 A19 A22 A24 A25 A27 A30 A33 A34 A37 A38 A40 A49 A51 A52 A55 A56 A59 A62 A64 A65 A72 A74 A76 A78 A81 A82 A85 A86 A88 L187 A90 A91 A96 A101 A102 A103 | S0 S3 L0 S5 S6 L2 L45 S8 S9 L46 S10 S11 L47 L158 L180 A22 L187 L191 | L0 L112 L113 L114 L115 L179 L180 L181 L182 A97 A99 A100 A101 A102 A103 | L0 L47 L113 L180 | L0 L112 L113 L114 L115 A97 A99 A100 | L0 L47 L112 L113 | L45 S8 S9 L46 S10 S11 L47 L51 S16 S17 L52 S18 S19 L53 L180 L191 | L47 L53 L112 L113 L179 L180 A98 | L0 L47 L112 L179 | L47 L112 L113 A98 | L49 L51 S16 S17 L52 S18 S19 L53 S20 S21 L54 S22 S23 L55 L57 S24 S25 L58 S26 S27 L59 S28 S29 L60 S30 S31 L179 L180 L183 L184 A94 A104 L189 L191 | L53 L179 L180 A104 | L0 L47 L179 L184 | L47 L53 L179 L184 | L147 L148 L149 L150 L151 L152 L153 L154 L155 L156 L157 L158 A17 A19 A22 A24 A25 A27 A30 A33 A34 A37 A38 A40 L187 | L158 A22 L187 | L0 L136 L137 L138 L139 L183 L184 L185 L186 A89 A90 A91 A92 A95 A96 | L0 L47 L136 L184 | L47 L53 L136 L139 L183 L184 A93 | L53 L183 L184 A94 | L0 L136 L137 L138 L139 A89 A92 A95 | L0 L47 L136 L139 | L43 L47 S12 S13 L48 S14 S15 L49 L53 S20 S21 L54 S22 S23 L166 L167 L183 A69 L189 | L1 L8 L9 L93 L94 L95 A9 A10 A11 A13 L187 L190 | L93 L94 L95 L140 L141 L142 A9 A10 A11 A12 A13 A14 A15 A16 | L0 L47 L139 L183 | L47 L136 L139 A93 | L0 S4 S7 L3 L47 S12 S13 L48 L167 L183 | L42 L43 L44 L45 L187 L189 L190 L191 | L1 L8 L9 L42 L187 L190 | L43 L44 L45 L49 L50 L51 L189 L191 | L49 L50 L51 L55 L56 L57 L188 L189 L191 | S1 S2 L3 L43 L48 S14 S15 L165 L166 A67 L187 L189 | L3 L48 L166 L167 | L48 L166 L167 A69 | L3 L159 L160 L161 L162 L163 L164 L165 L166 L167 L168 L169 L170 L171 L172 L173 L174 L175 L176 L177 L178 A49 A51 A52 A55 A56 A59 A62 A64 A65 A72 A74 A76 A78 A81 A82 A85 A86 A88 L187 | L165 L166 A67 L187 | S1 S2 L3 L166 L187 | L4 L5 L6 L7 | A4 | A5 | A6 | A7 | L10 L11 L18 L19 L20 L21 L22 L23 L24 L25 L26 L27 L28 L29 L30 L31 L32 L33 L67 L68 | L12 L13 L14 L15 L16 L17 L61 L62 L63 L64 L65 L66 | L34 L35 L36 L37 | L38 L39 L40 L41 | A8 | L96 L97 L98 L99 A41 A42 A46 A47 | L100 L101 L102 L103 L104 L105 L106 L107 L108 L109 L110 L111 A18 A20 A21 A23 A26 A28 A29 A31 A32 A35 A36 A39 | L116 L117 L118 L119 L120 L121 L122 L123 L124 L125 L126 L127 L128 L129 L130 L131 L132 L133 L134 L135 A50 A53 A54 A57 A58 A60 A61 A63 A66 A68 A70 A71 A73 A75 A77 A79 A80 A83 A84 A87 | L143 L144 L145 L146 A43 A44 A45 A48 makes body 1
ref_plane "WorkPlane8" through (182, 64.0022, 2) normal (0, 0, 1) x (1, 0, 0)
extrude "Extrude15" add sketch "triplejump-brd" along normal blind 0.5 from surface at 2 separate body contours L45 S8 S9 L46 S10 S11 L47 L51 S16 S17 L52 S18 S19 L53 L180 L191 | L47 L53 L112 L113 L179 L180 A98 | L47 L112 L113 A98 | L49 L51 S16 S17 L52 S18 S19 L53 S20 S21 L54 S22 S23 L55 L57 S24 S25 L58 S26 S27 L59 S28 S29 L60 S30 S31 L179 L180 L183 L184 A94 A104 L189 L191 | L53 L179 L180 A104 | L47 L53 L179 L184 | L47 L53 L136 L139 L183 L184 A93 | L53 L183 L184 A94 | L43 L47 S12 S13 L48 S14 S15 L49 L53 S20 S21 L54 S22 S23 L166 L167 L183 A69 L189 | L47 L136 L139 A93 | L43 L44 L45 L49 L50 L51 L189 L191 | L49 L50 L51 L55 L56 L57 L188 L189 L191 | L48 L166 L167 A69 | A4 | A5 | A6 | A7 | A8 makes body 2 at (19.8271, 14.7616, 2) makes body 3 at (237, 4.3355, 2) makes body 4 at (349.8271, 11.2384, 2) makes body 5 at (179.2976, 52.9747, 2) makes body 6 at (346.8879, 111.6709, 2) makes body 7 at (19.8271, 116.7617, 2)
ref_plane "WorkPlane9" through (17, 13, 2.5) normal (0, 0, 1) x (1, 0, 0)
extrude "Extrude16" add sketch "triplejump-brd" along normal blind 2.5 from surface at 2.5 separate body contours L45 S8 S9 L46 S10 S11 L47 L51 S16 S17 L52 S18 S19 L53 L180 L191 | L47 L53 L112 L113 L179 L180 A98 | L47 L112 L113 A98 | L49 L51 S16 S17 L52 S18 S19 L53 S20 S21 L54 S22 S23 L55 L57 S24 S25 L58 S26 S27 L59 S28 S29 L60 S30 S31 L179 L180 L183 L184 A94 A104 L189 L191 | L53 L179 L180 A104 | L47 L53 L179 L184 | L47 L53 L136 L139 L183 L184 A93 | L53 L183 L184 A94 | L43 L47 S12 S13 L48 S14 S15 L49 L53 S20 S21 L54 S22 S23 L166 L167 L183 A69 L189 | L47 L136 L139 A93 | L43 L44 L45 L49 L50 L51 L189 L191 | L49 L50 L51 L55 L56 L57 L188 L189 L191 | L48 L166 L167 A69 | A4 | A5 | A6 | A7 | A8 | L69 L70 L71 L72 L73 L74 | L75 L76 L77 L78 L79 L80 | L81 L82 L83 L84 L85 L86 | L87 L88 L89 L90 L91 L92 makes body 8 at (349.9776, 16.374, 4.1667) makes body 9 at (344.0224, 111.626, 4.1667) makes body 10 at (186.4944, 52.9029, 4.1667) makes body 11 at (237, 4.3355, 2.5) makes body 12 at (21.4944, 114.7757, 4.1667) makes body 13 at (21.4944, 12.7757, 4.1667)
ref_plane "WorkPlane10" through (17, 13, 5) normal (0, 0, 1) x (1, 0, 0)
extrude "Extrude17" add sketch "triplejump-brd" along normal blind 0.5 from surface at 2 separate body contours L93 L94 L95 L140 L141 L142 A9 A10 A11 A12 A13 A14 A15 A16 | L143 L144 L145 L146 A43 A44 A45 A48 makes body 14 at (172.6667, 105.1689, 2.5) makes body 15 at (136.6854, 104.7251, 2)
extrude "Extrude18" add sketch "triplejump-brd" along normal blind 2.5 from surface at 2.5 separate body contours L93 L94 L95 L140 L141 L142 A9 A10 A11 A12 A13 A14 A15 A16 | L143 L144 L145 L146 A43 A44 A45 A48 makes body 16 at (172.6667, 105.1689, 5) makes body 17 at (136.6854, 104.7251, 2.5)
extrude "Extrude19" add sketch "triplejump-brd" along normal blind 1.6 from surface at 5 separate body contours L45 S8 S9 L46 S10 S11 L47 L51 S16 S17 L52 S18 S19 L53 L180 L191 | L47 L53 L112 L113 L179 L180 A98 | L47 L112 L113 A98 | L47 L53 L179 L184 | L47 L53 L136 L139 L183 L184 A93 | L43 L47 S12 S13 L48 S14 S15 L49 L53 S20 S21 L54 S22 S23 L166 L167 L183 A69 L189 | L47 L136 L139 A93 | L43 L44 L45 L49 L50 L51 L189 L191 | L48 L166 L167 A69 makes body 18
ref_plane "WorkPlane11" through (182, 64.0022, 6.6) normal (0, 0, 1) x (1, 0, 0)
ref_plane "WorkPlane12" through (182, 64.0022, 10.6) normal (0, 0, 1) x (1, 0, 0)
ref_plane "WorkPlane13" through (182, 64.0022, 12.6) normal (0, 0, 1) x (1, 0, 0)
fillet "Fillet5" radius 1 12 edges at (350.8266, 124.2405, 0) (182, 125.0022, 0) (13.1734, 124.2405, 0) (7.7617, 118.8288, 0) (7, 64.0022, 0) (7.7617, 9.1756, 0) (13.1734, 3.7639, 0) (182, 3.0022, 0) (350.8266, 3.7639, 0) (356.2383, 9.1756, 0) (357, 64.0022, 0) (356.2383, 118.8288, 0) on bodies 1
extrude "Extrude1" [suppressed]
ref_plane "WorkPlane1" through (170, 56, 0.8) normal (0, 0, 1) x (1, 0, 0)
extrude "Extrude2" [suppressed]
ref_plane "WorkPlane2" through (170, 56, 4) normal (0, 0, 1) x (1, 0, 0)
extrude "Extrude3" [suppressed]
ref_plane "WorkPlane3" through (170, 56, 6.5) normal (0, 0, 1) x (1, 0, 0)
extrude "Extrude4" [suppressed]
extrude "Extrude5" [suppressed]
named bodies: "PCB", "b 2.0", "m b"
